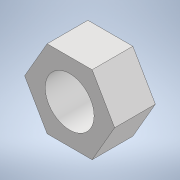
# Autodesk Inventor part: m6 Nut
Saved by Autodesk Inventor 2022 (Build 260153000, 153)
## iProperties
Created: 2022-05-05
Part Number: m6 Nut
Material: Generic
Document SubType Name: Modeling
Designer: erasm
Density: 1 g/cm^3
Appearance: Default
Author: erasm
Autodesk Inventor part; units mm, degrees
ref_plane "YZ Plane" through (0, 0, 0) normal (1, 0, 0) x (0, 1, 0)
ref_plane "XZ Plane" through (0, 0, 0) normal (0, 1, 0) x (-1, 0, 0)
ref_plane "XY Plane" through (0, 0, 0) normal (0, 0, 1) x (1, 0, 0)
sketch "Sketch1" plane through (0, 0, 0) normal (0, 0, 1) x (1, 0, 0)
  circle A0 centre (0, 0) radius 5.525
  line L0 (5.525, 0) -> (2.7625, -4.7848)
  line L1 (2.7625, -4.7848) -> (-2.7625, -4.7848)
  line L2 (-2.7625, -4.7848) -> (-5.525, 0)
  line L3 (-5.525, 0) -> (-2.7625, 4.7848)
  line L4 (-2.7625, 4.7848) -> (2.7625, 4.7848)
  line L5 (2.7625, 4.7848) -> (5.525, 0)
  circle A1 centre (0, 0) radius 3
  dimension "d0" = 11.05
  dimension "d1" = 6
  constraints: 12 end point, 2 coincident, 1 centre point, 1 horizontal alignment, 15 other
  measures "d1" diameter of A1
extrude "Extrusion1" add sketch "Sketch1" along normal blind 5 contours L0 L1 L2 L3 L4 L5
body "Solid1"
